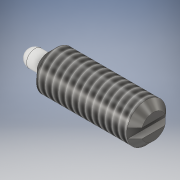
# Autodesk Inventor part: Spring_Separation
Saved by Autodesk Inventor 2018 (Build 220112000, 112)
## iProperties
Created: 2018-07-04
Part Number: Spring_Separation
Material: Stainless Steel
Document SubType Name: Modeling
Designer: Bradley
Density: 8 g/cm^3
Appearance: Semi-Polished
Author: Bradley
Autodesk Inventor part; units mm, degrees
ref_plane "YZ Plane" through (0, 0, 0) normal (1, 0, 0) x (0, 1, 0)
ref_plane "XZ Plane" through (0, 0, 0) normal (0, 1, 0) x (-1, 0, 0)
ref_plane "XY Plane" through (0, 0, 0) normal (0, 0, 1) x (1, 0, 0)
sketch "Sketch1" plane through (0, 0, 0) normal (0, 0, 1) x (1, 0, 0)
  line L0 (-6.7374, 0) -> (6.7374, 0)
  line L1 (6.7374, 0) -> (6.7374, 1.3208)
  line L2 (6.7374, 1.3208) -> (5.9754, 2.0828)
  line L3 (5.9754, 2.0828) -> (-3.6132, 2.0828)
  line L4 (-3.6132, 2.0828) -> (-4.3752, 1.3208)
  line L5 (-4.3752, 1.3208) -> (-4.3752, 0.889)
  line L6 (-4.3752, 0.889) -> (-5.8483, 0.889)
  arc A0 (-5.8483, 0.889) -> (-6.7374, 0) centre (-5.8483, 0) ccw
  point P0 (0, 0)
  point P1 (0, 0)
  dimension "d0" = 4.1656
  dimension "d1" = 11.1125
  dimension "d2" = 1.778
  dimension "d3" = 0.762
  dimension "d4" = 2.3622
  constraints: 14 end point, 4 perpendicular, 2 parallel, 2 point on circle, 1 centre point, 1 coincident, 1 horizontal, 1 horizontal alignment, 1 midpoint, 1 point on line, 1 tangent
  measures "d0" diameter of L3 L0
  measures "d1" distance between parallel lines of L1 L5
  measures "d2" diameter of L6 L0
  measures "d3" horizontal distance of L3.end L4.end
  measures "d4" distance from line of L5 L0.start
revolve "Revolution1" add sketch "Sketch1" angle 360 about axis through (-6.7374, 0, 0) along (1, 0, 0)
sketch "Sketch2" plane through (6.7374, 0, 0) normal (1, 0, 0) x (0, 0, -1)
  circle A0 centre (0, 0) radius 2.0828 projected
  circle A1 centre (0, 0) radius 1.3208 projected
  line L0 (-2.0828, 0.508) -> (2.0828, 0.508)
  line L1 (2.0828, 0.508) -> (2.0828, -0.508)
  line L2 (2.0828, -0.508) -> (-2.0828, -0.508)
  line L3 (-2.0828, -0.508) -> (-2.0828, 0.508)
  point P0 (0, 0)
  point P1 (-2.0828, 0)
  dimension "d6" = 1.016
  constraints: 8 end point, 2 parallel, 2 tangent, 1 horizontal, 1 horizontal alignment, 1 midpoint, 1 perpendicular
  measures "d6" distance of L2.end L0.start
extrude "Extrusion1" cut sketch "Sketch2" against normal blind 0.762 contours A0 L2 A1 L0 | L1 L2 A0 | A0 L0 L1 | L0 A1 L2 A0 | A0 L3 L0 | A1 L2 L0 | L2 L3 A0
thread "Thread1" size "8-36 UNF" class "2A" standard "ANSI Unified Screw Threads" full length
sketch "Sketch3" plane through (-4.3752, 0, 0) normal (-1, 0, 0) x (0, 0, 1)
  arc A0 (2.0199, -0.508) -> (2.0199, 0.508) centre (0, 0) ccw projected
  line L0 (-2.0199, -0.508) -> (2.0199, -0.508) projected
  arc A1 (-2.0199, 0.508) -> (-2.0199, -0.508) centre (0, 0) ccw projected
  line L1 (2.0199, 0.508) -> (-2.0199, 0.508) projected
  circle A2 centre (0, 0) radius 0.889 projected
  circle A3 centre (0, 0) radius 1.3208 projected
  arc A4 (-0.7296, 0.508) -> (-0.7296, -0.508) centre (0, 0) ccw
  arc A5 (0.7296, -0.508) -> (0.7296, 0.508) centre (0, 0) ccw
  point P0 (0, 0)
  constraints: 8 point on circle, 4 point on line, 2 centre point, 2 concentric
extrude "Extrusion2" cut sketch "Sketch3" against normal blind 0.762 contours L0 A3 L1 A0 | L0 A2 L1 A3 | A3 L1 A2 L0 | L0 A1 L1 A3
body "Solid1"
